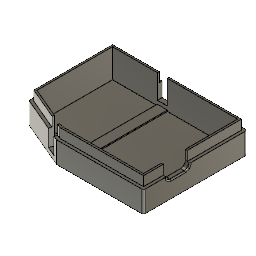
Boitier_Thermocouple_V1 (Autodesk Fusion 360 design; units mm, degrees)
Autodesk Fusion 360 part; units mm, degrees
sketch "Esquisse1" plane through (0, 0, 0) normal (0, 0, 1) x (1, 0, 0)
  line L0 (0, 0) -> (73, 0)
  line L1 (73, 0) -> (73, 87)
  line L2 (73, 87) -> (-40, 87)
  line L3 (-40, 87) -> (-40, 17)
  line L4 (-40, 17) -> (0, 0)
  dimension "d5" = 87
  dimension "d6" = 113
  dimension "d7" = 70
  dimension "d8" = 73
  constraint coincident L0.start L4.end
  constraint horizontal L0
  constraint perpendicular L0 L1
  constraint perpendicular L1 L2
  constraint perpendicular L2 L3
  measures "d5" distance of L0.end L1.end
  measures "d6" distance of L1.end L2.end
  measures "d7" distance of L2.end L3.end
  measures "d8" distance of L0.start L0.end
extrude "Extrusion1" add sketch "Esquisse1" along normal blind 3
sketch "Esquisse2" plane through (0, 0, 3) normal (0, 0, 1) x (-1, 0, 0)
  line L0 (40, -17) -> (0, 0)
  line L1 (0, 0) -> (-73, 0)
  line L2 (-73, 0) -> (-73, -87)
  line L3 (-73, -87) -> (40, -87)
  line L4 (40, -87) -> (40, -17)
  line L5 (-0.8147, -4) -> (-69, -4)
  line L6 (-69, -4) -> (-69, -83)
  line L7 (-69, -83) -> (36, -83)
  line L8 (36, -83) -> (36, -19.6463)
  line L9 (36, -19.6463) -> (-0.8147, -4)
  dimension "d11" = 4
  dimension "d12" = 4
  dimension "d13" = 4
  dimension "d14" = 4
  dimension "d15" = 4
  constraint horizontal L5
  constraint perpendicular L5 L6
  constraint perpendicular L6 L7
  constraint perpendicular L7 L8
  constraint parallel L0 L9
  measures "d11" distance of L2 L6
  measures "d12" distance of L3 L7
  measures "d13" distance of L4 L8
  measures "d14" distance of L1 L5
  measures "d15" distance of L0 L9
extrude "Extrusion2" add sketch "Esquisse2" along normal blind 15
sketch "Esquisse3" plane through (0, 0, 18) normal (0, 0, 1) x (-1, 0, 0)
  line L0 (-0.8147, -4) -> (36, -19.6463)
  line L1 (36, -19.6463) -> (36, -83)
  line L2 (36, -83) -> (-69, -83)
  line L3 (-69, -83) -> (-69, -4)
  line L4 (-69, -4) -> (-0.8147, -4)
  line L5 (40, -87) -> (40, -17)
  line L6 (40, -17) -> (0, 0)
  line L7 (0, 0) -> (-73, 0)
  line L8 (-73, 0) -> (-73, -87)
  line L9 (-73, -87) -> (40, -87)
  line L10 (37.6, -84.6) -> (-70.6, -84.6)
  line L11 (-70.6, -84.6) -> (-70.6, -2.4)
  line L12 (-70.6, -2.4) -> (-0.4888, -2.4)
  line L13 (-0.4888, -2.4) -> (37.6, -18.5878)
  line L14 (37.6, -18.5878) -> (37.6, -84.6)
  dimension "d18" = 1.6
  dimension "d19" = 1.6
  dimension "d20" = 1.6
  dimension "d21" = 1.6
  dimension "d22" = 1.6
  constraint parallel L2 L10
  constraint perpendicular L10 L11
  constraint perpendicular L11 L12
  constraint parallel L0 L13
  constraint parallel L1 L14
  measures "d18" distance of L2 L10
  measures "d19" distance of L3 L11
  measures "d20" distance of L4 L12
  measures "d21" distance of L0 L13
  measures "d22" distance of L1 L14
extrude "Extrusion3" add sketch "Esquisse3" along normal blind 8 contours L10 L11 L12 L13 L14
sketch "Esquisse4" plane through (0, 0, 3) normal (0, 0, 1) x (-1, 0, 0)
  line L0 (-0.8147, -4) -> (-69, -4)
  line L1 (-69, -4) -> (-69, -83)
  line L2 (-69, -83) -> (36, -83)
  line L3 (36, -83) -> (36, -19.6463)
  line L4 (36, -19.6463) -> (-0.8147, -4)
  line L5 (-69, -83) -> (-10, -83)
  line L6 (-10, -83) -> (-10, -4)
  line L7 (-10, -4) -> (-69, -4)
  line L8 (-69, -4) -> (-69, -83)
  line L9 (36, -83) -> (-1.5, -83)
  line L10 (-1.5, -83) -> (-1.5, -19.6463)
  line L11 (-1.5, -19.6463) -> (36, -19.6463)
  line L12 (36, -19.6463) -> (36, -83)
  dimension "d25" = 59
  dimension "d27" = 37.5
  constraint horizontal L5
  constraint vertical L6
  constraint horizontal L7
  constraint vertical L8
  constraint coincident L0 L6.end
  constraint coincident L1.end L2.start
  constraint horizontal L9
  constraint vertical L10
  constraint horizontal L11
  constraint vertical L12
  constraint coincident L2.end L3.start
  constraint coincident L3.end L4.start
  measures "d25" distance of L6 L8
  measures "d27" distance of L10 L12
extrude "Extrusion4" cut sketch "Esquisse4" against normal blind 1 contours L0 L1 L2 L5 L6 L7 L8 | L2 L3 L9 L10 L11 L12
sketch "Esquisse5" plane through (73, 0, 0) normal (1, 0, 0) x (0, 1, 0)
  line L0 (0, 0) -> (87, 0)
  line L1 (87, 0) -> (87, 18)
  line L2 (87, 18) -> (0, 18)
  line L3 (0, 18) -> (0, 0)
  line L4 (23, 14) -> (35, 14)
  arc A0 (35, 14) -> (35, 22) centre (35, 18) ccw
  line L5 (35, 22) -> (23, 22)
  arc A1 (23, 22) -> (23, 14) centre (23, 18) ccw
  line L6 (19, 18) -> (39, 18)
  line L7 (39, 18) -> (39, 26)
  line L8 (39, 26) -> (19, 26)
  line L9 (19, 26) -> (19, 18)
  line L10 (2.4, 26) -> (84.6, 26)
  dimension "d34" = 8
  dimension "d35" = 12
  dimension "d36" = 23
  dimension "d37" = 14
  dimension "d38" = 4
  constraint parallel L2 L4
  constraint tangent L4 A0
  constraint tangent A0 L5
  constraint parallel L4 L5
  constraint tangent L5 A1
  constraint horizontal L6
  constraint vertical L7
  constraint horizontal L8
  constraint vertical L9
  constraint coincident A1 L6.start
  constraint coincident L2 L6.start
  constraint coincident A0 L6.end
  constraint collinear L8 L10
  measures "d34" distance of L4 L5
  measures "d35" horizontal distance of A0.centre A1.centre
  measures "d36" distance of L3 A1.centre
  measures "d37" distance of L0 L4
  measures "d38" radius of A1
extrude "Extrusion5" cut sketch "Esquisse5" against normal blind 5 contours L2 A0 L5 A1 L6 | A0 L5 A1 L7 L8 L9 L10 | L2 L4 A0 A1 L6
sketch "Esquisse10" plane through (1.5646, 3.6813, 0) normal (0.391141, 0.920331, 0) x (-0.920331, 0.391141, 0)
  line L0 (0.8147, 3) -> (40.8164, 3)
  line L1 (40.8164, 3) -> (40.8164, 26)
  line L2 (40.8164, 26) -> (0.8147, 26)
  line L3 (0.8147, 26) -> (0.8147, 3)
  line L4 (3.8147, 26) -> (12.8147, 26)
  line L5 (12.8147, 26) -> (12.8147, 4)
  line L6 (12.8147, 4) -> (3.8147, 4)
  line L7 (3.8147, 4) -> (3.8147, 26)
  dimension "d55" = 9
  dimension "d56" = 22
  dimension "d57" = 3
  constraint horizontal L4
  constraint vertical L5
  constraint horizontal L6
  constraint vertical L7
  constraint collinear L2 L4
  measures "d55" distance of L4.start L4.end
  measures "d56" distance of L4.end L5.end
  measures "d57" distance of L3 L7
extrude "Extrusion8" cut sketch "Esquisse10" against normal blind 5 contours L2 L4 L5 L6 L7
sketch "Esquisse11" plane through (0, 83, 0) normal (0, -1, 0) x (1, 0, 0)
  line L0 (69, 2) -> (69, 26)
  line L1 (69, 26) -> (-36, 26)
  line L2 (-36, 26) -> (-36, 2)
  line L3 (1.5, 2) -> (1.5, 3)
  line L4 (1.5, 3) -> (10, 3)
  line L5 (10, 3) -> (10, 2)
  line L6 (9.8, 26) -> (1.7, 26)
  line L7 (1.7, 26) -> (1.7, 6)
  line L8 (1.7, 6) -> (9.8, 6)
  line L9 (9.8, 6) -> (9.8, 26)
  line L10 (-36, 2) -> (1.5, 2)
  line L11 (10, 2) -> (69, 2)
  dimension "d60" = 8.1
  dimension "d61" = 20
  dimension "d62" = 0.2
  constraint horizontal L6
  constraint vertical L7
  constraint horizontal L8
  constraint vertical L9
  constraint coincident L1 L6.start
  measures "d60" distance of L7.end L8.end
  measures "d61" distance of L6.start L8.end
  measures "d62" distance of L3.end L7
extrude "Extrusion9" cut sketch "Esquisse11" against normal blind 5 contours L1 L6 L7 L8 L9
fillet "Congé1" radius 2 5 edges at (0, 0, 9) (73, 0, 9) (-40, 17, 9) (73, 87, 9) (-40, 87, 9)
fillet "Congé2" radius 1 2 edges at (-17.5926, 11.8231, 3) (5.4074, 4, 3)
fillet "Congé3" radius 1 3 edges at (73, 37.8284, 15.1716) (73, 29, 14) (73, 20.1716, 15.1716)
equation "d16 = 20 mm - 5 mm"
